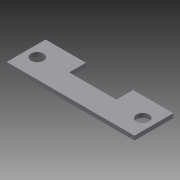
# Autodesk Inventor part: MotorBar
Saved by Autodesk Inventor 2014 SP1 (Build 180222100, 222)
## iProperties
Created: 2015-03-30
Part Number: MotorBar
Material: Generic
Document SubType Name: Modeling
Designer: Erin
Density: 1 g/cm^3
Appearance: Default
Author: Erin
Autodesk Inventor part; units mm, degrees
ref_plane "YZ Plane" through (0, 0, 0) normal (1, 0, 0) x (0, 1, 0)
ref_plane "XZ Plane" through (0, 0, 0) normal (0, 1, 0) x (-1, 0, 0)
ref_plane "XY Plane" through (0, 0, 0) normal (0, 0, 1) x (1, 0, 0)
sketch "Sketch1" plane through (0, 0, 0) normal (0, 0, 1) x (1, 0, 0)
  line L0 (-15, 7) -> (15, 7)
  line L1 (15, 7) -> (15, -7)
  line L2 (15, -7) -> (-15, -7)
  line L3 (-15, -7) -> (-15, 7)
  line L4 (-15, 7) -> (-23, 7)
  line L5 (-23, 7) -> (-23, -7)
  line L6 (-23, -7) -> (-15, -7)
  line L7 (-15, -7) -> (-15, 7)
  line L8 (15, 7) -> (23, 7)
  line L9 (23, 7) -> (23, -7)
  line L10 (23, -7) -> (15, -7)
  line L11 (15, -7) -> (15, 7)
  line L12 (-23, 0) -> (23, 0) construction
  circle A0 centre (-19, 0) radius 2.25
  circle A1 centre (19, 0) radius 2.25
  line L13 (0, 7) -> (0, -7) construction
  line L14 (-8.5, 7) -> (8.5, 7)
  line L15 (8.5, 7) -> (8.5, 1)
  line L16 (8.5, 1) -> (-8.5, 1)
  line L17 (-8.5, 1) -> (-8.5, 7)
  point P0 (0, 0)
  point P1 (0, 0)
  point P2 (0, 7)
  point P3 (0, 0)
  dimension "d0" = 14
  dimension "d1" = 30
  dimension "d2" = 4.5
  dimension "d3" = 4.5
  dimension "d4" = 4
  dimension "d5" = 4
  dimension "d6" = 4
  dimension "d7" = 4
  dimension "d10" = 17
  dimension "d11" = 6
  constraints: 36 end point, 8 parallel, 7 midpoint, 5 horizontal, 4 perpendicular, 3 point on line, 2 centre point, 1 coincident, 1 collinear, 1 vertical alignment
  measures "d0" distance of L2.end L0.start
  measures "d1" distance of L0.start L0.end
  measures "d2" diameter of A0
  measures "d3" diameter of A1
  measures "d4" distance from line of A1.centre L9
  measures "d5" distance from line of A1.centre L1
  measures "d6" distance from line of A0.centre L5
  measures "d7" distance from line of A0.centre L3
  measures "d10" distance of L15.end L16.end
  measures "d11" distance of L14.end L15.end
extrude "Extrusion1" add sketch "Sketch1" along normal blind 1.5 contours L0 L17 L16 L15 L1 L2 L3 | L3 L6 L5 L4 | L1 L8 L9 L10
body "Solid1"
